Autodesk Fusion 360 part; units mm, degrees
(part 2 of 2)
sketch "Sketch20" plane through (0, 0, 0) normal (0, 0, -1) x (1, 0, 0)
  line L0 (50, 0) -> (50, -5)
  line L1 (50, -5) -> (40, -5)
  line L2 (40, -5) -> (40, 0)
  line L3 (40, 0) -> (30, 0)
  line L4 (30, 0) -> (30, -5)
  line L5 (30, -5) -> (20, -5)
  line L6 (20, -5) -> (20, 0)
  line L7 (20, 0) -> (10, 0)
  line L8 (10, 0) -> (10, -5)
  line L9 (10, -5) -> (5, -5)
  line L10 (5, -5) -> (5, -10)
  line L11 (5, -10) -> (0, -10)
  line L12 (0, -10) -> (0, -20)
  line L13 (0, -20) -> (5, -20)
  line L14 (5, -20) -> (5, -30)
  line L15 (5, -30) -> (0, -30)
  line L16 (0, -30) -> (0, -40)
  line L17 (0, -40) -> (5, -40)
  line L18 (5, -40) -> (5, -50)
  line L19 (5, -50) -> (0, -50)
  line L20 (0, -50) -> (0, -60)
  line L21 (0, -60) -> (5, -60)
  line L22 (5, -60) -> (5, -70)
  line L23 (5, -70) -> (0, -70)
  line L24 (0, -70) -> (0, -80)
  line L25 (0, -80) -> (5, -80)
  line L26 (5, -80) -> (5, -85)
  line L27 (5, -85) -> (10, -85)
  line L28 (10, -85) -> (10, -90)
  line L29 (10, -90) -> (20, -90)
  line L30 (20, -90) -> (20, -85)
  line L31 (20, -85) -> (30, -85)
  line L32 (30, -85) -> (30, -90)
  line L33 (30, -90) -> (40, -90)
  line L34 (40, -90) -> (40, -85)
  line L35 (40, -85) -> (50, -85)
  line L36 (50, -85) -> (50, -90)
  line L37 (50, -90) -> (60, -90)
  line L38 (60, -90) -> (60, -85)
  line L39 (60, -85) -> (70, -85)
  line L40 (70, -85) -> (70, -90)
  line L41 (70, -90) -> (80, -90)
  line L42 (80, -90) -> (80, -85)
  line L43 (80, -85) -> (85, -85)
  line L44 (85, -85) -> (85, -80)
  line L45 (85, -80) -> (90, -80)
  line L46 (90, -80) -> (90, -70)
  line L47 (90, -70) -> (85, -70)
  line L48 (85, -70) -> (85, -60)
  line L49 (85, -60) -> (90, -60)
  line L50 (90, -60) -> (90, -50)
  line L51 (90, -50) -> (85, -50)
  line L52 (85, -50) -> (85, -40)
  line L53 (85, -40) -> (90, -40)
  line L54 (90, -40) -> (90, -30)
  line L55 (90, -30) -> (85, -30)
  line L56 (85, -30) -> (85, -20)
  line L57 (85, -20) -> (90, -20)
  line L58 (90, -20) -> (90, -10)
  line L59 (90, -10) -> (85, -10)
  line L60 (85, -10) -> (85, -5)
  line L61 (85, -5) -> (80, -5)
  line L62 (80, -5) -> (80, 0)
  line L63 (80, 0) -> (70, 0)
  line L64 (70, 0) -> (70, -5)
  line L65 (70, -5) -> (60, -5)
  line L66 (60, -5) -> (60, 0)
  line L67 (60, 0) -> (50, 0)
sketch "Sketch21" plane through (0, 0, 50) normal (0, 0, 1) x (-1, 0, 0)
  circle A0 centre (-76.5099, -13.4901) radius 3
  circle A1 centre (-76.5099, -76.5099) radius 3
  circle A2 centre (-13.4901, -76.5099) radius 3
  circle A3 centre (-13.4901, -13.4901) radius 3
  circle A4 centre (-45, -45) radius 17.5
  line L0 (-50, -5) -> (-50, 0)
  line L1 (-50, 0) -> (-60, 0)
  line L2 (-60, 0) -> (-60, -5)
  line L3 (-60, -5) -> (-70, -5)
  line L4 (-70, -5) -> (-70, 0)
  line L5 (-70, 0) -> (-80, 0)
  line L6 (-80, 0) -> (-80, -5)
  line L7 (-80, -5) -> (-85, -5)
  line L8 (-85, -5) -> (-85, -10)
  line L9 (-85, -10) -> (-90, -10)
  line L10 (-90, -10) -> (-90, -20)
  line L11 (-90, -20) -> (-85, -20)
  line L12 (-85, -20) -> (-85, -30)
  line L13 (-85, -30) -> (-90, -30)
  line L14 (-90, -30) -> (-90, -40)
  line L15 (-90, -40) -> (-85, -40)
  line L16 (-85, -40) -> (-85, -50)
  line L17 (-85, -50) -> (-90, -50)
  line L18 (-90, -50) -> (-90, -60)
  line L19 (-90, -60) -> (-85, -60)
  line L20 (-85, -60) -> (-85, -70)
  line L21 (-85, -70) -> (-90, -70)
  line L22 (-90, -70) -> (-90, -80)
  line L23 (-90, -80) -> (-85, -80)
  line L24 (-85, -80) -> (-85, -85)
  line L25 (-85, -85) -> (-80, -85)
  line L26 (-80, -85) -> (-80, -90)
  line L27 (-80, -90) -> (-70, -90)
  line L28 (-70, -90) -> (-70, -85)
  line L29 (-70, -85) -> (-60, -85)
  line L30 (-60, -85) -> (-60, -90)
  line L31 (-60, -90) -> (-50, -90)
  line L32 (-50, -90) -> (-50, -85)
  line L33 (-50, -85) -> (-40, -85)
  line L34 (-40, -85) -> (-40, -90)
  line L35 (-40, -90) -> (-30, -90)
  line L36 (-30, -90) -> (-30, -85)
  line L37 (-30, -85) -> (-20, -85)
  line L38 (-20, -85) -> (-20, -90)
  line L39 (-20, -90) -> (-10, -90)
  line L40 (-10, -90) -> (-10, -85)
  line L41 (-10, -85) -> (-5, -85)
  line L42 (-5, -85) -> (-5, -80)
  line L43 (-5, -80) -> (0, -80)
  line L44 (0, -80) -> (0, -70)
  line L45 (0, -70) -> (-5, -70)
  line L46 (-5, -70) -> (-5, -60)
  line L47 (-5, -60) -> (0, -60)
  line L48 (0, -60) -> (0, -50)
  line L49 (0, -50) -> (-5, -50)
  line L50 (-5, -50) -> (-5, -40)
  line L51 (-5, -40) -> (0, -40)
  line L52 (0, -40) -> (0, -30)
  line L53 (0, -30) -> (-5, -30)
  line L54 (-5, -30) -> (-5, -20)
  line L55 (-5, -20) -> (0, -20)
  line L56 (0, -20) -> (0, -10)
  line L57 (0, -10) -> (-5, -10)
  line L58 (-5, -10) -> (-5, -5)
  line L59 (-5, -5) -> (-10, -5)
  line L60 (-10, -5) -> (-10, 0)
  line L61 (-10, 0) -> (-20, 0)
  line L62 (-20, 0) -> (-20, -5)
  line L63 (-20, -5) -> (-30, -5)
  line L64 (-30, -5) -> (-30, 0)
  line L65 (-30, 0) -> (-40, 0)
  line L66 (-40, 0) -> (-40, -5)
  line L67 (-40, -5) -> (-50, -5)
component "Component" placed x (1, 0, 0) y (0, 1, 0) z (0, 0, 1) at (0, 0, 0)
component "Component'" placed x (1, 0, 0) y (0, 1, 0) z (0, 0, 1) at (0, 0, 0)
